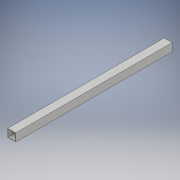
# Autodesk Inventor part: LateralBars
Saved by Autodesk Inventor 2019.3 (Build 233278000, 278)
## iProperties
Created: 2019-06-25
Part Number: LateralBars
Material: Generic
Document SubType Name: Modeling
Designer: mark
Density: 1 g/cm^3
Appearance: Default
Author: mark
Autodesk Inventor part; units mm, degrees
ref_plane "YZ Plane" through (0, 0, 0) normal (1, 0, 0) x (0, 1, 0)
ref_plane "XZ Plane" through (0, 0, 0) normal (0, 1, 0) x (-1, 0, 0)
ref_plane "XY Plane" through (0, 0, 0) normal (0, 0, 1) x (1, 0, 0)
sketch "Sketch1" plane through (0, 0, 0) normal (0, 0, 1) x (1, 0, 0)
  line L0 (93.1, 0) -> (67.7, 0) projected
  line L1 (93.1, 0) -> (67.7, 0) projected
  line L2 (10, 0) -> (35.4, 0)
  line L3 (35.4, 0) -> (35.4, 25.4)
  line L4 (35.4, 25.4) -> (10, 25.4)
  line L5 (10, 25.4) -> (10, 0)
  line L6 (11.5875, 1.5875) -> (33.8125, 1.5875)
  line L7 (33.8125, 1.5875) -> (33.8125, 23.8125)
  line L8 (33.8125, 23.8125) -> (11.5875, 23.8125)
  line L9 (11.5875, 23.8125) -> (11.5875, 1.5875)
  line L10 (67.7, 25.4) -> (67.7, 0) projected
  line L11 (93.1, 0) -> (93.1, 25.4) projected
  line L12 (93.1, 25.4) -> (67.7, 25.4) projected
  line L13 (67.7, 25.4) -> (67.7, 0) projected
  line L14 (93.1, 0) -> (93.1, 25.4) projected
  line L15 (93.1, 25.4) -> (67.7, 25.4) projected
  point P0 (0, 0)
  dimension "d0" = 22.225
  dimension "d1" = 22.225
  dimension "d3" = 1.5875
  constraints: 16 end point, 1 parallel
  measures "d0" distance between parallel lines of L8 L6
  measures "d1" distance between parallel lines of L7 L9
  measures "d3" distance between parallel lines of L6 L0
extrude "Extrusion1" add sketch "Sketch1" along normal blind 500 contours L5 L4 L3 L2
body "Solid1"
